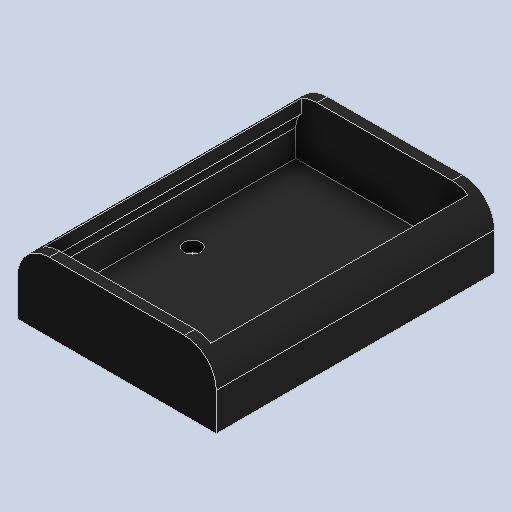
# Autodesk Inventor part: battery_box
Saved by Autodesk Inventor 2026.1 (Build 301233020, 233B)
## iProperties
Created: 2026-01-22
Part Number: battery_box
Material: 一般
Document SubType Name: Modeling
Designer: hibik
Density: 1 g/cm^3
Appearance: 既定
Author: hibik
Autodesk Inventor part; units mm, degrees
ref_plane "YZ Plane" through (0, 0, 0) normal (1, 0, 0) x (0, 1, 0)
ref_plane "XZ Plane" through (0, 0, 0) normal (0, 1, 0) x (-1, 0, 0)
ref_plane "XY Plane" through (0, 0, 0) normal (0, 0, 1) x (1, 0, 0)
sketch "スケッチ1" plane through (0, 0, 0) normal (0, 1, 0) x (-1, 0, 0)
  line L0 (-18.75, -26.25) -> (18.75, -26.25)
  line L1 (18.75, -26.25) -> (18.75, 26.25)
  line L2 (18.75, 26.25) -> (-18.75, 26.25)
  line L3 (-18.75, 26.25) -> (-18.75, -26.25)
  line L4 (-18.75, -26.25) -> (18.75, 26.25) construction
  line L5 (18.75, -26.25) -> (-18.75, 26.25) construction
  point P0 (0, 0)
  dimension "d0" = 37.5
  dimension "d1" = 52.5
  constraints: 12 end point, 2 midpoint, 2 parallel, 1 horizontal, 1 perpendicular
  measures "d0" distance of L2.end L1.end
  measures "d1" distance of L1.end L0.end
extrude "押し出し1" add sketch "スケッチ1" along normal blind 13.1
fillet "フィレット1" radius 6 2 edges at (18.75, 13.1, 0) (-18.75, 13.1, 0)
shell "シェル1" thickness 2 removed faces 0
sketch "スケッチ2" plane through (0, 13.1, 0) normal (0, 1, 0) x (1, 0, 0)
  line L0 (16.75, 24.25) -> (-16.75, 24.25) projected
  line L1 (15.75, -24.25) -> (-15.75, -24.25)
  line L2 (-15.75, -24.25) -> (-15.75, 24.25)
  line L3 (-15.75, 24.25) -> (15.75, 24.25)
  line L4 (15.75, 24.25) -> (15.75, -24.25)
  line L5 (15.75, -24.25) -> (-15.75, 24.25) construction
  line L6 (-15.75, -24.25) -> (15.75, 24.25) construction
  line L7 (-12.75, -26.25) -> (-12.75, 26.25) projected
  point P0 (0, 0)
  dimension "d8" = 3
  constraints: 12 end point, 2 midpoint, 2 parallel, 1 horizontal, 1 perpendicular, 1 point on line
  measures "d8" distance between parallel lines of L7 L2
extrude "押し出し2" cut sketch "スケッチ2" against normal blind 5
sketch "スケッチ3" plane through (-16.75, 2, 24.25) normal (0, 1, 0) x (1, 0, 0)
  circle A0 centre (28.75, 24.25) radius 1.6
  circle A1 centre (4.75, 24.25) radius 1.6
  line L0 (4, 48.5) -> (29.5, 48.5) projected
  line L1 (16.75, 48.5) -> (16.75, 0) construction
  line L2 (0, 0) -> (33.5, 0) projected
  point P0 (16.75, 24.25)
  dimension "d9" = 3.2
  dimension "d11" = 24
  constraints: 2 centre point, 2 end point, 2 midpoint, 1 horizontal alignment, 1 other
  measures "d9" diameter of A0
  measures "d11" distance of A0.centre A1.centre
extrude "押し出し3" cut sketch "スケッチ3" against normal through all
